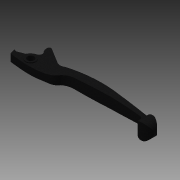
# Autodesk Inventor part: MAN
Saved by Autodesk Inventor 2016 (Build 200138000, 138)
## iProperties
Created: 2013-07-10
Part Number: MAN
Material: Generic
Document SubType Name: Modeling
Designer: Luis
Density: 1 g/cm^3
Appearance: Fine Textured - Black
Author: Luis
Autodesk Inventor part; units mm, degrees
ref_plane "YZ Plane" through (0, 0, 0) normal (1, 0, 0) x (0, 1, 0)
ref_plane "XZ Plane" through (0, 0, 0) normal (0, 1, 0) x (-1, 0, 0)
ref_plane "XY Plane" through (0, 0, 0) normal (0, 0, 1) x (1, 0, 0)
sketch "Sketch1" plane through (0, 0, 0) normal (0, 0, 1) x (1, 0, 0)
  line L0 (545.1177, -659.7811) -> (543.1172, -653.1128)
  line L1 (543.1172, -653.1128) -> (546.3933, -653.954)
  line L2 (546.8648, -653.9286) -> (555.3753, -650.7372)
  line L3 (565.5906, -628.3557) -> (585.29, -640.4612)
  line L4 (661.6824, -638.3842) -> (701.382, -642.1863)
  line L5 (701.382, -642.1863) -> (711.1668, -643.438)
  line L6 (711.1668, -643.438) -> (714.7071, -645.0396)
  line L7 (697.1659, -646.9866) -> (684.2309, -646.5188)
  line L8 (684.2309, -646.5188) -> (659.2401, -646.2281)
  line L9 (659.2401, -646.2281) -> (613.5494, -648.0763)
  arc A0 (545.1177, -659.7811) -> (545.4566, -660.0594) centre (545.4941, -659.6682) ccw
  arc A1 (546.3933, -653.954) -> (546.8648, -653.9286) centre (546.5888, -653.1927) ccw
  arc A2 (562.8823, -644.3706) -> (555.3753, -650.7372) centre (565.7536, -655.3653) ccw
  arc A3 (562.8823, -644.3706) -> (565.5906, -638.384) centre (561.5138, -640.1457) ccw
  arc A4 (562.5496, -630.2746) -> (565.5906, -638.384) centre (571.5807, -631.5129) ccw
  arc A5 (565.5906, -628.3557) -> (562.5496, -630.2746) centre (565.1403, -631.0112) ccw
  arc A6 (585.29, -640.4612) -> (594.8583, -640.8073) centre (590.3971, -631.706) ccw
  arc A7 (661.6824, -638.3842) -> (594.8583, -640.8073) centre (635.5259, -839.6851) ccw
  arc A8 (719.4278, -650.2259) -> (714.7071, -645.0396) centre (711.4064, -652.7856) ccw
  arc A9 (714.7071, -656.5151) -> (719.4278, -650.2259) centre (710.637, -648.5438) ccw
  arc A10 (704.6273, -657.7797) -> (714.7071, -656.5151) centre (708.1369, -644.9496) ccw
  arc A11 (700.0188, -651.2301) -> (704.6273, -657.7797) centre (707.1824, -651.0857) ccw
  arc A12 (700.0188, -651.2301) -> (697.1659, -646.9866) centre (695.2949, -651.3253) ccw
  arc A13 (613.5494, -648.0763) -> (601.6075, -653.0719) centre (614.3004, -666.6428) ccw
  arc A14 (592.5304, -659.3266) -> (601.6075, -653.0719) centre (590.6768, -646.9227) ccw
  arc A15 (566.2399, -662.0499) -> (592.5304, -659.3266) centre (570.8255, -578.0544) ccw
  arc A16 (545.4566, -660.0594) -> (566.2399, -662.0499) centre (580.1428, -407.3877) ccw
  circle A17 centre (564.3151, -653.5334) radius 4.2463
  point P0 (0, 0)
  dimension "d30" = 0.393
  dimension "d31" = 0.786
  constraints: 34 point on circle, 20 end point, 18 centre point, 6 tangent
  measures "d30" radius of A0
  measures "d31" radius of A1
extrude "Extrusion1" add sketch "Sketch1" along normal blind 20
sketch "Sketch2" plane through (0, 0, 0) normal (0, 1, 0) x (-1, 0, 0)
  line L0 (-543.1172, 0) -> (-543.1172, 20) projected
  line L1 (-700.0198, 5.5) -> (-700.0198, 14.5)
  line L2 (-543.1172, 5.5) -> (-543.1172, 14.5)
  line L3 (-700.0198, 10) -> (-543.1172, 10) construction
  line L4 (-621.5685, 10) -> (-621.5685, 3.5) construction
  line L5 (-543.1172, 5.5) -> (-586.8527, 5.5)
  arc A0 (-698.8271, 5.3992) -> (-589.3495, 5.3959) centre (-644.0685, 660.5736) ccw
  arc A1 (-586.8527, 5.5) -> (-589.3495, 5.3959) centre (-586.8527, -24.5) ccw
  line L6 (-543.1172, 14.5) -> (-586.8527, 14.5)
  arc A2 (-589.3495, 14.6041) -> (-698.8271, 14.6008) centre (-644.0685, -640.5736) ccw
  arc A3 (-589.3495, 14.6041) -> (-586.8527, 14.5) centre (-586.8527, 44.5) ccw
  line L7 (-527.985, -16.5873) -> (-734.4622, -16.5873)
  line L8 (-734.4622, -16.5873) -> (-734.4622, 28.3783)
  line L9 (-734.4622, 28.3783) -> (-527.985, 28.3783)
  line L10 (-527.985, 28.3783) -> (-527.985, -16.5873)
  arc A4 (-700.6647, 15.4949) -> (-700.6647, 4.5051) centre (-709.0198, 10) ccw
  arc A5 (-698.8271, 5.3992) -> (-700.6647, 4.5051) centre (-698.9937, 3.4062) ccw
  arc A6 (-700.6647, 15.4949) -> (-698.8271, 14.6008) centre (-698.9937, 16.5938) ccw
  point P0 (0, 0)
  point P1 (0, 0)
  point P2 (0, 0)
  point P3 (-588.1172, 5.5)
  dimension "d42" = 9
  dimension "d43" = 9
  dimension "d45" = 6.5
  dimension "d46" = 45
  dimension "d47" = 30
  dimension "d48" = 20
  dimension "d49" = 9
  dimension "d50" = 2
  constraints: 20 end point, 18 point on circle, 7 centre point, 6 tangent, 4 midpoint, 4 parallel, 4 symmetric about line, 2 perpendicular, 2 point on line, 1 equal radius, 1 horizontal, 1 vertical, 4 other
  measures "d42" distance of L1.start L1.end
  measures "d43" distance of L2.start L2.end
  measures "d45" distance of L4.start L4.end
  measures "d46" distance of L2.start point (-588.117, 5.5)
  measures "d47" radius of A1
  measures "d48" diameter of A4
  measures "d49" distance of A4.centre L3.start
  measures "d50" radius of A5
extrude "Extrusion2" cut sketch "Sketch2" against normal through all
sketch "Sketch3" plane through (586.8527, -660.634, 14.5) normal (0, 0, 1) x (1, 0, 0)
  circle A0 centre (-22.5376, 7.1007) radius 4.2463 projected
  circle A1 centre (-22.5376, 7.1007) radius 6.5
  point P0 (-586.8527, 660.634)
  dimension "d53" = 13
  constraints: 1 centre point, 1 coincident
  measures "d53" diameter of A1
extrude "Extrusion3" add sketch "Sketch3" along normal blind 1
sketch "Sketch4" plane through (586.8527, -660.634, 5.5) normal (0, 0, -1) x (-1, 0, 0)
  circle A0 centre (22.5376, 7.1007) radius 4.2463 projected
  circle A1 centre (22.5376, 7.1007) radius 6.5
  point P0 (586.8527, 660.634)
  dimension "d56" = 13
  constraints: 1 centre point, 1 coincident
  measures "d56" diameter of A1
extrude "Extrusion4" add sketch "Sketch4" along normal blind 1
sketch "Sketch5" plane through (586.8527, -660.634, 5.5) normal (0, 0, -1) x (-1, 0, 0)
  line L0 (43.7354, 7.5213) -> (41.735, 0.8529) projected
  line L1 (0, 19.4321) -> (0, 0) projected
  line L2 (43.7354, 7.5213) -> (53.7354, 7.5213)
  line L3 (53.7354, 7.5213) -> (41.735, 0.8529)
  point P0 (586.8527, 660.634)
  dimension "d59" = 10
  constraints: 4 end point, 1 perpendicular
  measures "d59" distance of L0.start L2.end
extrude "Extrusion5" [suppressed]
fillet "Fillet1" [suppressed]
body "Solid1"
